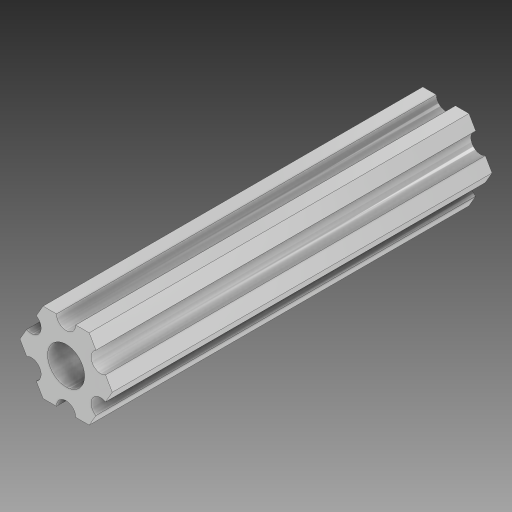
# Autodesk Inventor part: Configurable Kitbot Churro
Saved by Autodesk Inventor 2023 (Build 270158030, 158C)
## iProperties
Created: 2023-01-20
Part Number: Configurable Kitbot Churro
Material: Aluminum
Document SubType Name: Modeling
Designer: Max Boord
Density: 2.7 g/cm^3
Appearance: Aluminum - Dark
Author: Max Boord
Autodesk Inventor part; units mm, degrees
ref_plane "YZ Plane" through (0, 0, 0) normal (1, 0, 0) x (0, 1, 0)
ref_plane "XZ Plane" through (0, 0, 0) normal (0, 1, 0) x (-1, 0, 0)
ref_plane "XY Plane" through (0, 0, 0) normal (0, 0, 1) x (1, 0, 0)
sketch "Sketch1" plane through (0, 0, 0) normal (0, 0, 1) x (1, 0, 0)
  line L0 (-7.3323, 0) -> (-3.6662, 6.35)
  line L1 (-3.6662, 6.35) -> (3.6662, 6.35)
  line L2 (3.6662, 6.35) -> (7.3323, 0)
  line L3 (7.3323, 0) -> (3.6662, -6.35)
  line L4 (3.6662, -6.35) -> (-3.6662, -6.35)
  line L5 (-3.6662, -6.35) -> (-7.3323, 0)
  circle A0 centre (0, 6.35) radius 1.524
  circle A1 centre (-5.4993, 3.175) radius 1.524
  circle A2 centre (-5.4993, -3.175) radius 1.524
  circle A3 centre (0, -6.35) radius 1.524
  circle A4 centre (5.4993, -3.175) radius 1.524
  circle A5 centre (5.4993, 3.175) radius 1.524
  circle A6 centre (0, 0) radius 2.9337
  point P0 (6.2613, 1.8552)
  point P1 (4.7373, 4.4948)
  point P2 (1.524, 6.35)
  point P3 (-1.524, 6.35)
  point P4 (-4.7373, 4.4948)
  point P5 (-6.2613, 1.8552)
  point P6 (-6.2613, -1.8552)
  point P7 (-4.7373, -4.4948)
  point P8 (-1.524, -6.35)
  point P9 (1.524, -6.35)
  point P10 (4.7373, -4.4948)
  point P11 (6.2613, -1.8552)
  dimension "d0" = 12.7
  dimension "d1" = 3.048
  dimension "d4" = 360
  dimension "d6" = 5.8674
  constraints: 12 end point, 7 centre point, 2 coincident, 1 horizontal, 1 midpoint, 26 other
  measures "d0" distance between parallel lines of L4 L1
  measures "d1" diameter of A0
  measures "d6" diameter of A6
extrude "Extrusion1" add sketch "Sketch1" along normal mid plane 60.325 contours L0 A1 L1 A0 L2 A5 L3 A4 L4 A3 L5 A2
body "Solid1"
